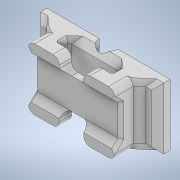
# Autodesk Inventor part: Cable Holder
Saved by Autodesk Inventor 2022 (Build 260153000, 153)
## iProperties
Created: 2021-04-23
Part Number: Cable Holder
Material: Generic
Document SubType Name: Modeling
Designer: Viktor
Density: 1 g/cm^3
Appearance: Default
Author: Viktor
## iProperties of the stored document Cable Holder_3DPrint.ipt
Created: 2021-04-23
Part Number: Cable Holder_3DPrint
Material: Generic
Document SubType Name: Modeling
Designer: Viktor
Density: 1 g/cm^3
Appearance: Default
Author: Viktor
Autodesk Inventor part; units mm, degrees
ref_plane "YZ Plane" through (0, 0, 0) normal (1, 0, 0) x (0, 1, 0)
ref_plane "XZ Plane" through (0, 0, 0) normal (0, 1, 0) x (-1, 0, 0)
ref_plane "XY Plane" through (0, 0, 0) normal (0, 0, 1) x (1, 0, 0)
sketch "Sketch1" plane through (0, 0, 0) normal (0, 0, 1) x (1, 0, 0)
  line L0 (-20, -10) -> (20, -10)
  line L1 (20, -10) -> (20, 10)
  line L2 (20, 10) -> (-20, 10)
  line L3 (-20, 10) -> (-20, -10)
  line L4 (-20, -10) -> (20, 10) construction
  line L5 (20, -10) -> (-20, 10) construction
  point P0 (0, 0)
  dimension "d0" = 20
  dimension "d1" = 40
  constraints: 12 end point, 2 midpoint, 2 parallel, 1 horizontal, 1 perpendicular
  measures "d0" distance between parallel lines of L0 L2
  measures "d1" distance between parallel lines of L1 L3
extrude "Extrusion1" add sketch "Sketch1" along normal blind 4
sketch "Sketch2" plane through (0, 0, 4) normal (0, 0, 1) x (1, 0, 0)
  line L0 (-14, -10) -> (14, -10)
  line L1 (14, -10) -> (14, 10)
  line L2 (14, 10) -> (-14, 10)
  line L3 (-14, 10) -> (-14, -10)
  line L4 (-14, -10) -> (14, 10) construction
  line L5 (14, -10) -> (-14, 10) construction
  point P0 (0, 0)
  constraints: 12 end point, 2 midpoint, 2 parallel, 1 horizontal, 1 perpendicular
extrude "Extrusion2" add sketch "Sketch2" along normal blind 8
sketch "Sketch3" plane through (14, -10, 4) normal (1, 0, 0) x (0, 0, -1)
  line L0 (-8, 0) -> (-8, 20) projected
  line L1 (-8, 0) -> (-8, 3)
  line L2 (-8, 3) -> (-6, 5)
  line L3 (-6, 5) -> (-6, 15)
  line L4 (-6, 15) -> (-8, 17)
  line L5 (-8, 20) -> (-8, 0) projected
  point P0 (4, 10)
  dimension "d6" = 3
  dimension "d7" = 3
  dimension "d8" = 135
  dimension "d9" = 135
  dimension "d10" = 2
  constraints: 8 end point, 2 point on line
  measures "d6" distance of L0.end L4.end
  measures "d7" distance of L1.end L0.start
  measures "d8" angle of L0 L2
  measures "d9" angle of L0 L4
  measures "d10" distance between parallel lines of L0 L3
extrude "Extrusion3" cut sketch "Sketch3" against normal through all
sketch "Sketch4" plane through (-20, -10, 0) normal (0, -1, 0) x (1, 0, 0)
  line L0 (34, 4) -> (34, 12) projected
  line L1 (6, 4) -> (34, 4)
  line L2 (34, 4) -> (34, 8)
  line L3 (34, 8) -> (6, 8)
  line L4 (6, 8) -> (6, 4)
  line L5 (6, 12) -> (34, 12) projected
  line L6 (10, 4) -> (30, 4)
  line L7 (30, 4) -> (30, 8)
  line L8 (30, 8) -> (10, 8)
  line L9 (10, 8) -> (10, 4)
  point P0 (20, 0)
  dimension "d13" = 4
  dimension "d14" = 4
  dimension "d15" = 4
  constraints: 16 end point, 4 parallel, 2 horizontal, 2 perpendicular, 2 point on line, 1 midpoint
  measures "d13" distance between parallel lines of L5 L3
  measures "d14" distance between parallel lines of L4 L9
  measures "d15" distance between parallel lines of L0 L7
extrude "Extrusion4" cut sketch "Sketch4" against normal through all contours L1 L9 L3 L7
sketch "Sketch5" plane through (-20, -10, 0) normal (0, -1, 0) x (1, 0, 0)
  line L0 (20, 14.4) -> (20, -2.4) projected
  line L1 (16, 8) -> (24, 8)
  line L2 (24, 8) -> (24, 12)
  line L3 (24, 12) -> (16, 12)
  line L4 (16, 12) -> (16, 8)
  line L5 (34, 10) -> (6, 10) projected
  line L6 (16, 8) -> (24, 12) construction
  line L7 (24, 8) -> (16, 12) construction
  point P0 (20, 0)
  point P1 (20, 10)
  dimension "d18" = 8
  constraints: 12 end point, 3 midpoint, 2 parallel, 1 horizontal, 1 perpendicular
  measures "d18" distance of L2.end L3.end
extrude "Extrusion5" cut sketch "Sketch5" against normal blind 5
mirror "Mirror1" about plane through (0, 0, 0) normal (0, 1, 0) of "Extrusion5"
fillet "Fillet1" radius 2 16 edges at (4, -10, 10) (-4, -10, 10) (-14, -10, 8) (14, -10, 8) (14, 10, 8) (-4, 10, 10) (4, 10, 10) (-4, 5, 9) (4, 5, 9) (4, -5, 9) (-4, -5, 9) (-14, 10, 8) (-10, 10, 6) (10, 10, 6) (10, -10, 6) (-10, -10, 6)
chamfer "Chamfer1" distance 2 angle 45 12 edges at (14, 0, 4) (13.4142, -9.4142, 4) (13.4142, 9.4142, 4) (-14, 0, 4) (-13.4142, 9.4142, 4) (-13.4142, -9.4142, 4) (10, 0, 4) (10, 0, 8) (-10, 0, 8) (-10.5858, 9.4142, 8) (-10, 0, 4) (-10.5858, 9.4142, 4)
chamfer "Chamfer2" distance 2 angle 45 3 edges at (-10, 0, 6) (-10.5858, 9.4142, 6) (10, 0, 6)
chamfer "Chamfer3" distance 1 angle 45 6 edges at (14, 0, 10) (-14, 0, 10) (-14, -6, 11) (-14, 6, 11) (14, -6, 11) (14, 6, 11)
chamfer "Chamfer4" distance 2 angle 45 8 edges at (-20, 0, 4) (20, 0, 4) (17.7321, -10, 4) (0, -10, 4) (-17.7321, -10, 4) (17.7321, 10, 4) (0, 10, 4) (-17.7321, 10, 4)
sketch "Sketch6" plane through (-20, 10, 0) normal (0, 1, 0) x (1, 0, 0)
  circle A0 centre (20, 0) radius 3
  dimension "d34" = 6
  constraints: 1 centre point, 1 coincident
  measures "d34" diameter of A0
extrude "Extrusion6" cut sketch "Sketch6" against normal through all
equation "\"d6\" = d7"
equation "\"d9\" = d8"
equation "\"d15\" = d14"
body "Solid1"
